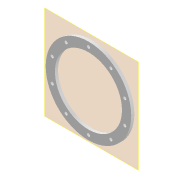
# Autodesk Inventor part: Anglerfish_3inch_tube_pressurering
Saved by Autodesk Inventor 2022 (Build 260153000, 153)
## iProperties
Created: 2022-04-17
Part Number: Anglerfish_3inch_tube_pressurering
Material: Generic
Document SubType Name: Modeling
Designer: Prakash Lab
Density: 1 g/cm^3
Appearance: Default
Author: Prakash Lab
Autodesk Inventor part; units mm, degrees
ref_plane "YZ Plane" through (0, 0, 0) normal (1, 0, 0) x (0, 1, 0)
ref_plane "XZ Plane" through (0, 0, 0) normal (0, 1, 0) x (-1, 0, 0)
ref_plane "XY Plane" through (0, 0, 0) normal (0, 0, 1) x (1, 0, 0)
ref_plane "Work Plane1" through (0, 0, 0) normal (0, 0, 1) x (1, 0, 0)
sketch "Sketch1" plane through (0, 0, 0) normal (0, 0, 1) x (1, 0, 0)
  circle A0 centre (-29.1541, -40.1272) radius 2 projected
  circle A1 centre (-47.1724, -15.3272) radius 2 projected
  circle A2 centre (-47.1724, 15.3272) radius 2 projected
  circle A3 centre (-29.1541, 40.1272) radius 2 projected
  circle A4 centre (0, 49.6) radius 2 projected
  circle A5 centre (29.1541, 40.1272) radius 2 projected
  circle A6 centre (47.1724, 15.3272) radius 2 projected
  circle A7 centre (47.1724, -15.3272) radius 2 projected
  circle A8 centre (29.1541, -40.1272) radius 2 projected
  circle A9 centre (0, -49.6) radius 2 projected
  circle A10 centre (0, 0) radius 55.6 projected
  circle A11 centre (0, 0) radius 43.6
  dimension "d0" = 12
  constraints: 1 centre point, 1 coincident
  measures "d0" radial gap between concentric circles of A11 A10
extrude "Extrusion1" add sketch "Sketch1" along normal blind 4
body "Solid1"
